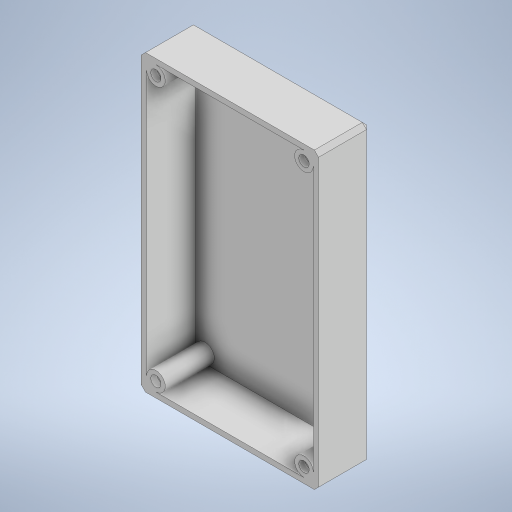
# Autodesk Inventor part: LV_Deckel
Saved by Autodesk Inventor 2024 (Build 280153000, 153)
## iProperties
Created: 2026-06-02
Part Number: LV_Deckel
Material: Generisch
Document SubType Name: Modeling
Designer: maxim
Density: 1 g/cm^3
Appearance: Vorgabe
Author: maxim
Autodesk Inventor part; units mm, degrees
ref_plane "YZ Plane" through (0, 0, 0) normal (1, 0, 0) x (0, 1, 0)
ref_plane "XZ Plane" through (0, 0, 0) normal (0, 1, 0) x (-1, 0, 0)
ref_plane "XY Plane" through (0, 0, 0) normal (0, 0, 1) x (1, 0, 0)
sketch "Skizze1" plane through (0, 0, 0) normal (0, 1, 0) x (-1, 0, 0)
  line L0 (0, 0) -> (0, -127)
  line L1 (0, -127) -> (71, -127)
  line L2 (71, -127) -> (71, 0)
  line L3 (71, 0) -> (0, 0)
  circle A0 centre (71, 0) radius 2.5
  circle A1 centre (71, -127) radius 2.5
  circle A2 centre (0, -127) radius 2.5
  circle A3 centre (0, 0) radius 2.5
  dimension "d0" = 127
  dimension "d1" = 71
  dimension "d2" = 5
  dimension "d3" = 5
  dimension "d4" = 5
  dimension "d5" = 5
  constraints: 8 end point, 4 centre point, 4 coincident, 2 parallel, 1 perpendicular, 1 vertical
  measures "d0" distance of L0.start L0.end
  measures "d1" distance of L1.end L0.end
  measures "d2" diameter of A0
  measures "d3" diameter of A1
  measures "d4" diameter of A2
  measures "d5" diameter of A3
sketch "Skizze2" plane through (0, 0, 0) normal (0, 1, 0) x (-1, 0, 0)
  line L0 (71, -127) -> (71, 0) projected
  line L1 (71, 0) -> (0, 0) projected
  line L2 (0, 0) -> (0, -127) projected
  line L3 (0, -127) -> (71, -127) projected
  line L4 (78, 7) -> (78, -134)
  line L5 (78, -134) -> (-7, -134)
  line L6 (-7, -134) -> (-7, 7)
  line L7 (-7, 7) -> (78, 7)
  dimension "d6" = 7
  constraints: 8 end point, 3 other
  measures "d6" distance between parallel lines of L0 L4
extrude "Extrusion1" add sketch "Skizze2" along normal blind 25 contours L3 L2 L1 L0 | L4 L5 L6 L7
extrude "Extrusion2" cut sketch "Skizze1" along normal blind 3 contours L3 A3 L0 | L0 A3 L3 | A2 L1 L0 | L0 L1 A2 | A0 L2 L3 | L3 L2 A0 | A1 L2 L1 | L1 L2 A1
sketch "Skizze3" plane through (0, 0, 0) normal (0, -1, 0) x (1, 0, 0)
  circle A0 centre (-71, -127) radius 2.5 projected
  circle A1 centre (-71, -127) radius 4.5
  circle A2 centre (-71, 0) radius 2.5 projected
  circle A3 centre (-71, 0) radius 4.5
  circle A4 centre (0, 0) radius 2.5 projected
  circle A5 centre (0, 0) radius 4.5
  circle A6 centre (0, -127) radius 2.5 projected
  circle A7 centre (0, -127) radius 4.5
  line L0 (-78, 7) -> (7, 7) projected
  line L1 (-78, -134) -> (-78, 7) projected
  line L2 (7, -134) -> (-78, -134) projected
  line L3 (7, 7) -> (7, -134) projected
  line L4 (-75.5, 4.5) -> (4.5, 4.5)
  line L5 (4.5, 4.5) -> (4.5, -131.5)
  line L6 (4.5, -131.5) -> (-75.5, -131.5)
  line L7 (-75.5, -131.5) -> (-75.5, 4.5)
  point P0 (-35.5, 7)
  point P1 (-78, -63.5)
  point P2 (-75.5, 0)
  point P3 (-75.5, -127)
  point P4 (-71, -131.5)
  point P5 (0, -131.5)
  point P6 (4.5, -127)
  point P7 (4.5, 0)
  point P8 (0, 4.5)
  point P9 (-71, 4.5)
  dimension "d11" = 9
  dimension "d12" = 9
  dimension "d13" = 9
  dimension "d14" = 9
  constraints: 8 end point, 4 centre point, 4 coincident, 2 midpoint, 1 tangent, 3 other
  measures "d11" diameter of A1
  measures "d12" diameter of A3
  measures "d13" diameter of A5
  measures "d14" diameter of A7
extrude "Extrusion3" cut sketch "Skizze3" against normal blind 23.5 contours A1 L7 A3 L4 A5 L5 A7 L6
chamfer "Fasen1" distance 2 angle 45 8 edges at (-78, 12.5, -134) (-78, 12.5, 7) (7, 12.5, -134) (7, 12.5, 7) (7, 25, -63.5) (-35.5, 25, 7) (-78, 25, -63.5) (-35.5, 25, -134)
